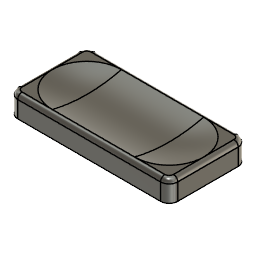
koiboard (Autodesk Fusion 360 archive; units mm, degrees)
design "keycap 2u"
part number: 2026-03-29-00-46-45-191
Autodesk Fusion 360 part; units mm, degrees
sketch "Sketch1" plane through (0, 0, 0) normal (0, 0, 1) x (1, 0, 0)
  line L0 (0, 0) -> (37.05, 0)
  line L1 (37.05, 0) -> (37.05, -18)
  line L2 (37.05, -18) -> (0, -18)
  line L3 (0, -18) -> (0, 0)
  line L4 (21.025, -10.3) -> (16.025, -10.3)
  line L5 (16.025, -10.3) -> (16.025, -7.7)
  line L6 (16.025, -7.7) -> (21.025, -7.7)
  line L7 (21.025, -7.7) -> (21.025, -10.3)
  line L8 (21.025, -10.3) -> (16.025, -7.7) construction
  line L9 (16.025, -10.3) -> (21.025, -7.7) construction
  line L10 (20.625, -9.6) -> (16.425, -9.6)
  line L11 (16.425, -9.6) -> (16.425, -8.4)
  line L12 (16.425, -8.4) -> (20.625, -8.4)
  line L13 (20.625, -8.4) -> (20.625, -9.6)
  line L14 (20.625, -9.6) -> (16.425, -8.4) construction
  line L15 (16.425, -9.6) -> (20.625, -8.4) construction
  line L16 (17.225, -6.5) -> (19.825, -11.5) construction
  line L17 (17.925, -11.1) -> (19.125, -6.9) construction
  line L18 (17.225, -11.5) -> (19.825, -6.5) construction
  line L19 (17.225, -6.5) -> (19.825, -6.5)
  line L20 (17.925, -11.1) -> (17.925, -6.9)
  line L21 (17.225, -11.5) -> (17.225, -6.5)
  line L22 (17.925, -6.9) -> (19.125, -11.1) construction
  line L23 (19.825, -6.5) -> (19.825, -11.5)
  line L24 (19.825, -11.5) -> (17.225, -11.5)
  line L25 (19.125, -6.9) -> (19.125, -11.1)
  line L26 (19.125, -11.1) -> (17.925, -11.1)
  line L27 (17.925, -6.9) -> (19.125, -6.9)
  line L28 (36.35, -0.7) -> (0.7, -0.7)
  line L29 (0.7, -0.7) -> (0.7, -17.3)
  line L30 (0.7, -17.3) -> (36.35, -17.3)
  line L31 (36.35, -17.3) -> (36.35, -0.7)
  point P0 (18.525, -9)
  point P1 (18.525, -9)
  point P2 (18.525, -9)
  point P3 (18.525, -9)
  point P4 (18.525, -9)
  point P5 (18.525, -9)
  dimension "d1" = 37.05
  dimension "d2" = 18
  dimension "d9" = 5
  dimension "d10" = 2.6
  dimension "d11" = 4.2
  dimension "d12" = 1.2
  dimension "d13" = 5
  dimension "d14" = 2.6
  dimension "d15" = 4.2
  dimension "d16" = 1.2
  dimension "d21" = 35.65
  dimension "d22" = 16.6
  constraint horizontal L0
  constraint vertical L1
  constraint horizontal L2
  constraint vertical L3
  constraint coincident L0.start L3.end
  constraint horizontal L4
  constraint perpendicular L4 L5
  constraint parallel L4 L6
  constraint parallel L5 L7
  constraint coincident L8 P5
  constraint coincident L9 P5
  constraint horizontal L10
  constraint perpendicular L10 L11
  constraint parallel L10 L12
  constraint parallel L11 L13
  constraint coincident L14 P5
  constraint coincident L15 P5
  constraint coincident P5 P4
  constraint perpendicular L19 L21
  constraint parallel L21 L23
  constraint parallel L19 L24
  constraint coincident P5 L18
  constraint coincident P5 L16
  constraint perpendicular L20 L27
  constraint parallel L20 L25
  constraint parallel L26 L27
  constraint coincident P5 L17
  constraint coincident P5 L22
  constraint horizontal L28
  constraint perpendicular L28 L29
  constraint parallel L29 L31
  measures "d1" distance of L0.start L0.end
  measures "d2" distance of L0.start L2.end
  measures "d9" distance of L5.end L6.end
  measures "d10" distance of L4.end L5.end
  measures "d11" distance of L11.end L12.end
  measures "d12" distance of L10.end L11.end
  measures "d13" distance of L18.end L16.end
  measures "d14" distance of L18.end L16.start
  measures "d15" distance of L22.end L17.end
  measures "d16" distance of L20.end L17.end
  measures "d21" distance of L29.end L30.end
  measures "d22" distance of L28.end L29.end
extrude "Extrude1" add sketch "Sketch1" along normal blind 4.9 contours L0 L1 L2 L3 | L4 L6 L7 L10 L12 L13 L23 | L4 L20 L21 L23 L24 L25 L26 | L4 L10 L23 L25 | L4 L20 L25 L26 | L4 L10 L20 L25 | L10 L12 L13 L23 | L10 L12 L23 L25 | L6 L12 L23 L25 | L6 L19 L20 L21 L23 L25 L27 | L4 L10 L20 L21 | L10 L12 L20 L25 | L6 L12 L20 L25 | L6 L20 L25 L27 | L4 L5 L6 L10 L11 L12 L21 | L10 L12 L20 L21 | L6 L12 L20 L21 | L10 L11 L12 L21 | L28 L29 L30 L31
fillet "Fillet1" radius 2 4 edges at (37.05, -18, 2.45) (37.05, 0, 2.45) (0, 0, 2.45) (0, -18, 2.45)
extrude "Extrude2" cut sketch "Sketch1" along normal blind 3.4 contours L4 L6 L7 L10 L12 L13 L23 | L4 L20 L21 L23 L24 L25 L26 | L4 L10 L23 L25 | L4 L20 L25 L26 | L4 L10 L20 L25 | L10 L12 L13 L23 | L10 L12 L23 L25 | L6 L12 L23 L25 | L6 L19 L20 L21 L23 L25 L27 | L4 L10 L20 L21 | L10 L12 L20 L25 | L6 L12 L20 L25 | L6 L20 L25 L27 | L4 L5 L6 L10 L11 L12 L21 | L10 L12 L20 L21 | L6 L12 L20 L21 | L10 L11 L12 L21 | L28 L29 L30 L31
fillet "Fillet2" radius 1.3 4 edges at (36.35, -17.3, 1.7) (0.7, -17.3, 1.7) (0.7, -0.7, 1.7) (36.35, -0.7, 1.7)
extrude "Extrude3" add sketch "Sketch1" along normal blind 5 from surface at -1 contours L4 L6 L7 L10 L12 L13 L23 | L4 L20 L21 L23 L24 L25 L26 | L4 L10 L23 L25 | L6 L12 L23 L25 | L6 L19 L20 L21 L23 L25 L27 | L4 L10 L20 L21 | L4 L5 L6 L10 L11 L12 L21 | L6 L12 L20 L21
fillet "Fillet3" radius 0.5 8 edges at (19.825, -11.5, 1.2) (21.025, -10.3, 1.2) (21.025, -7.7, 1.2) (19.825, -6.5, 1.2) (17.225, -6.5, 1.2) (16.025, -7.7, 1.2) (16.025, -10.3, 1.2) (17.225, -11.5, 1.2)
ref_plane "WorkPlane1" through (0, 0, 36.4) normal (0, 0, 1) x (1, 0, 0)
sketch "Sketch2" plane through (0, 0, 36.4) normal (0, 0, 1) x (1, 0, 0)
  point P0 (9, -9)
  point P1 (28.05, -9)
sphere "SpherePrimitive1" cut diameter 65 placed x (1, 0, 0) y (0, 1, 0) z (0, 0, 1) at (9, -9, 36.4)
fillet "Fillet4" radius 1 8 edges at (36.4642, -17.4142, 4.9) (37.05, -9, 4.9) (36.4642, -0.5858, 4.9) (18.525, 0, 4.9) (0.5858, -0.5858, 4.9) (0, -9, 4.9) (0.5858, -17.4142, 4.9) (18.525, -18, 4.9)
sphere "SpherePrimitive2" cut diameter 65 placed x (1, 0, 0) y (0, 1, 0) z (0, 0, 1) at (28.05, -9, 36.4)
ref_plane "WorkPlane4" through (9, 0, 0) normal (1, 0, 0) x (0, 1, 0)
cylinder "CylinderPrimitive1" cut diameter 65 height 19.05 placed x (0, 0, -1) y (0, 1, 0) z (1, 0, 0) at (9, -9, 36.4)
equation "d1 = 18 mm + 18 mm + ( 19.05 mm - 18 mm )"
equation "d21 = 37.05 mm - 1.4 mm"
equation "d22 = 18 mm - 1.4 mm"
equation "d23 = 4.9 mm - ( 4.9 mm - 3.4 mm )"
equation "d32 = 31.5 mm + 4.9 mm"
equation "d40 = ( 18 mm + 18 mm - ( 19.05 mm - 18 mm ) - 8 mm - 8 mm ) + 0.1 mm"

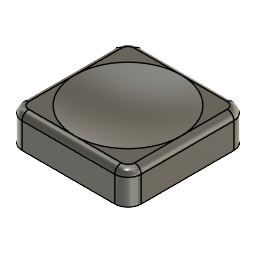
design "keycap"
part number: 2026-03-29-00-46-45-191
Autodesk Fusion 360 part; units mm, degrees
sketch "Sketch1" plane through (0, 0, 0) normal (0, 0, 1) x (1, 0, 0)
  line L0 (0, 0) -> (18, 0)
  line L1 (18, 0) -> (18, -18)
  line L2 (18, -18) -> (0, -18)
  line L3 (0, -18) -> (0, 0)
  line L4 (11.5, -10.3) -> (6.5, -10.3)
  line L5 (6.5, -10.3) -> (6.5, -7.7)
  line L6 (6.5, -7.7) -> (11.5, -7.7)
  line L7 (11.5, -7.7) -> (11.5, -10.3)
  line L8 (11.5, -10.3) -> (6.5, -7.7) construction
  line L9 (6.5, -10.3) -> (11.5, -7.7) construction
  line L10 (11.1, -9.6) -> (6.9, -9.6)
  line L11 (6.9, -9.6) -> (6.9, -8.4)
  line L12 (6.9, -8.4) -> (11.1, -8.4)
  line L13 (11.1, -8.4) -> (11.1, -9.6)
  line L14 (11.1, -9.6) -> (6.9, -8.4) construction
  line L15 (6.9, -9.6) -> (11.1, -8.4) construction
  line L16 (7.7, -6.5) -> (10.3, -11.5) construction
  line L17 (8.4, -11.1) -> (9.6, -6.9) construction
  line L18 (7.7, -11.5) -> (10.3, -6.5) construction
  line L19 (7.7, -6.5) -> (10.3, -6.5)
  line L20 (8.4, -11.1) -> (8.4, -6.9)
  line L21 (7.7, -11.5) -> (7.7, -6.5)
  line L22 (8.4, -6.9) -> (9.6, -11.1) construction
  line L23 (10.3, -6.5) -> (10.3, -11.5)
  line L24 (10.3, -11.5) -> (7.7, -11.5)
  line L25 (9.6, -6.9) -> (9.6, -11.1)
  line L26 (9.6, -11.1) -> (8.4, -11.1)
  line L27 (8.4, -6.9) -> (9.6, -6.9)
  line L28 (17.3, -0.7) -> (0.7, -0.7)
  line L29 (0.7, -0.7) -> (0.7, -17.3)
  line L30 (0.7, -17.3) -> (17.3, -17.3)
  line L31 (17.3, -17.3) -> (17.3, -0.7)
  line L32 (17.3, -0.7) -> (0.7, -17.3) construction
  line L33 (0.7, -0.7) -> (17.3, -17.3) construction
  point P0 (9, -9)
  point P1 (9, -9)
  point P2 (9, -9)
  point P3 (9, -9)
  point P4 (9, -9)
  dimension "d1" = 18
  dimension "d2" = 18
  dimension "d9" = 5
  dimension "d10" = 2.6
  dimension "d11" = 4.2
  dimension "d12" = 1.2
  dimension "d13" = 5
  dimension "d14" = 2.6
  dimension "d15" = 4.2
  dimension "d16" = 1.2
  dimension "d21" = 16.6
  dimension "d22" = 16.6
  constraint horizontal L0
  constraint vertical L1
  constraint horizontal L2
  constraint vertical L3
  constraint coincident L0.start L3.end
  constraint horizontal L4
  constraint perpendicular L4 L5
  constraint parallel L4 L6
  constraint parallel L5 L7
  constraint coincident L8 P4
  constraint coincident L9 P4
  constraint horizontal L10
  constraint perpendicular L10 L11
  constraint parallel L10 L12
  constraint parallel L11 L13
  constraint coincident L14 P4
  constraint coincident L15 P4
  constraint coincident P4 P3
  constraint perpendicular L19 L21
  constraint parallel L21 L23
  constraint parallel L19 L24
  constraint coincident P4 L18
  constraint coincident P4 L16
  constraint perpendicular L20 L27
  constraint parallel L20 L25
  constraint parallel L26 L27
  constraint coincident P4 L17
  constraint coincident P4 L22
  constraint horizontal L28
  constraint perpendicular L28 L29
  constraint parallel L28 L30
  constraint parallel L29 L31
  constraint coincident L32 P4
  constraint coincident L33 P4
  measures "d1" distance of L0.start L0.end
  measures "d2" distance of L0.start L2.end
  measures "d9" distance of L5.end L6.end
  measures "d10" distance of L4.end L5.end
  measures "d11" distance of L11.end L12.end
  measures "d12" distance of L10.end L11.end
  measures "d13" distance of L18.end L16.end
  measures "d14" distance of L18.end L16.start
  measures "d15" distance of L22.end L17.end
  measures "d16" distance of L20.end L17.end
  measures "d21" distance of L29.end L30.end
  measures "d22" distance of L28.end L29.end
extrude "Extrude1" add sketch "Sketch1" along normal blind 4.9 contours L0 L1 L2 L3 | L4 L6 L7 L10 L12 L13 L23 | L4 L20 L21 L23 L24 L25 L26 | L4 L10 L23 L25 | L4 L20 L25 L26 | L4 L10 L20 L25 | L10 L12 L13 L23 | L10 L12 L23 L25 | L6 L12 L23 L25 | L6 L19 L20 L21 L23 L25 L27 | L4 L10 L20 L21 | L10 L12 L20 L25 | L6 L12 L20 L25 | L6 L20 L25 L27 | L4 L5 L6 L10 L11 L12 L21 | L10 L12 L20 L21 | L6 L12 L20 L21 | L10 L11 L12 L21 | L28 L29 L30 L31
fillet "Fillet1" radius 2 4 edges at (18, -18, 2.45) (18, 0, 2.45) (0, 0, 2.45) (0, -18, 2.45)
extrude "Extrude2" cut sketch "Sketch1" along normal blind 3.4 contours L4 L6 L7 L10 L12 L13 L23 | L4 L20 L21 L23 L24 L25 L26 | L4 L10 L23 L25 | L4 L20 L25 L26 | L4 L10 L20 L25 | L10 L12 L13 L23 | L10 L12 L23 L25 | L6 L12 L23 L25 | L6 L19 L20 L21 L23 L25 L27 | L4 L10 L20 L21 | L10 L12 L20 L25 | L6 L12 L20 L25 | L6 L20 L25 L27 | L4 L5 L6 L10 L11 L12 L21 | L10 L12 L20 L21 | L6 L12 L20 L21 | L10 L11 L12 L21 | L28 L29 L30 L31
fillet "Fillet2" radius 1.3 4 edges at (17.3, -17.3, 1.7) (0.7, -17.3, 1.7) (0.7, -0.7, 1.7) (17.3, -0.7, 1.7)
extrude "Extrude3" add sketch "Sketch1" along normal blind 5 from surface at -1 contours L4 L6 L7 L10 L12 L13 L23 | L4 L20 L21 L23 L24 L25 L26 | L4 L10 L23 L25 | L6 L12 L23 L25 | L6 L19 L20 L21 L23 L25 L27 | L4 L10 L20 L21 | L4 L5 L6 L10 L11 L12 L21 | L6 L12 L20 L21
fillet "Fillet3" radius 0.5 8 edges at (10.3, -11.5, 1.2) (11.5, -10.3, 1.2) (11.5, -7.7, 1.2) (10.3, -6.5, 1.2) (7.7, -6.5, 1.2) (6.5, -7.7, 1.2) (6.5, -10.3, 1.2) (7.7, -11.5, 1.2)
ref_plane "WorkPlane1" through (0, 0, 36.4) normal (0, 0, 1) x (1, 0, 0)
sketch "Sketch2" plane through (0, 0, 36.4) normal (0, 0, 1) x (1, 0, 0)
  point P0 (9, -9)
sphere "SpherePrimitive1" cut diameter 65 placed x (1, 0, 0) y (0, 1, 0) z (0, 0, 1) at (9, -9, 36.4)
fillet "Fillet4" radius 1 8 edges at (17.4142, -17.4142, 4.9) (18, -9, 4.9) (17.4142, -0.5858, 4.9) (9, 0, 4.9) (0.5858, -0.5858, 4.9) (0, -9, 4.9) (0.5858, -17.4142, 4.9) (9, -18, 4.9)
equation "d21 = 18 mm - 1.4 mm"
equation "d22 = 18 mm - 1.4 mm"
equation "d23 = 4.9 mm - ( 4.9 mm - 3.4 mm )"
equation "d32 = 31.5 mm + 4.9 mm"

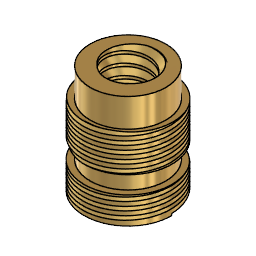
design "M2*4*3.2 insert"
part number: 2026-03-29-14-28-17-945
Autodesk Fusion 360 part; units mm, degrees
sketch "Sketch1" plane through (0, 0, 0) normal (0, 0, 1) x (1, 0, 0)
  circle A0 centre (5, 5) radius 1.4
  circle A1 centre (5, 5) radius 1.625
  circle A2 centre (5, 5) radius 0.75
  dimension "d1" = 2.8
  dimension "d2" = 3.25
  dimension "d10" = 1.5
  constraint concentric A0 A1
  constraint concentric A0 A2
  measures "d1" diameter of A0
  measures "d2" diameter of A1
  measures "d10" diameter of A2
extrude "Extrude1" add sketch "Sketch1" along normal blind 4 contours A0 | A2
extrude "Extrude2" add sketch "Sketch1" along normal blind 1 contours A1
extrude "Extrude3" add sketch "Sketch1" along normal blind 1.3 from surface at 1.65 contours A1
extrude "Extrude4" cut sketch "Sketch1" along normal blind 4 contours A2
thread "Thread1" "ISO Metric profile 2.0 M2x0.4 M2x0.4 6H" major diameter 2.074 minor diameter 1.623 pitch 0.4 angle 60 modelled right hand crest width 0.1065 on face at (5.7491, 4.9626, 2.6667) crest through (5.8115, 5, 0.1)
coil "CoilPrimitive1" cut diameter 3.4 section triangle in size 0.4 on centre turns 10.33333 pitch 0.3 right hand placed x (1, 0, 0) y (0, 1, 0) z (0, 0, 1) at (5, 5, 0)
